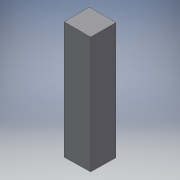
# Autodesk Inventor part: braço_junta_2
Saved by Autodesk Inventor 2018 (Build 220112000, 112)
## iProperties
Created: 2018-05-17
Part Number: braço_junta_2
Material: Genérico
Document SubType Name: Modeling
Designer: Usuario
Density: 1 g/cm^3
Appearance: Padrão
Author: Usuario
Autodesk Inventor part; units mm, degrees
ref_plane "YZ Plane" through (0, 0, 0) normal (1, 0, 0) x (0, 1, 0)
ref_plane "XZ Plane" through (0, 0, 0) normal (0, 1, 0) x (-1, 0, 0)
ref_plane "XY Plane" through (0, 0, 0) normal (0, 0, 1) x (1, 0, 0)
sketch "Esboço1" plane through (0, 0, 0) normal (0, 0, 1) x (1, 0, 0)
  line L0 (40, 339.6477) -> (0, 339.6477) projected
  line L1 (0, 339.6477) -> (40, 339.6477)
  line L2 (40, 339.6477) -> (40, 377.6477)
  line L3 (40, 377.6477) -> (0, 377.6477)
  line L4 (0, 377.6477) -> (0, 339.6477)
  line L5 (0, 377.6477) -> (65, 377.6477) construction
  point P0 (0, 0)
  dimension "d0" = 38
  constraints: 10 end point, 2 horizontal, 2 parallel, 1 perpendicular, 2 other
  measures "d0" distance of L2.end L1.end
ref_plane "Plano de trabalho1" through (-15.8286, 339.6534, -176.6311) normal (-0.0197852, 0.0122576, 0.9997291) x (0.9997606, 0.0095824, 0.0196683)
extrude "Extrusão1" add sketch "Esboço1" against normal up to surface surface through (-15.8286, 339.6534, -176.6311) normal (-0.0197852, 0.0122576, 0.9997291)
sketch "Esboço2" plane through (40, 339.6477, -175.5261) normal (0.0197852, -0.0122576, -0.9997291) x (-0.9998042, 0, -0.0197867)
  ellipse E0 centre (19.2853, 28.552) end of major axis (17.1791, 31.9526) minor radius 3.9989 construction
  ellipse E1 centre (19.2853, 9.5534) end of major axis (17.1791, 12.954) minor radius 3.9989 construction
  line L0 (40.0078, 0) -> (40.0171, 38.0029) construction
  line L1 (40.0124, 19.0014) -> (0.0046, 19.0014) construction
  line L2 (0.0092, 38.0029) -> (0, 0) construction
  line L3 (40.0171, 38.0029) -> (0.0092, 38.0029) construction
  line L4 (20.0131, 38.0029) -> (20.0039, 0) construction
  line L5 (0, 0) -> (40.0078, 0) construction
  line L6 (20.0085, 19.0014) -> (20.011, 29.0014) construction
  line L7 (20.0085, 19.0014) -> (20.0061, 9.0014) construction
  point P0 (36.5191, -341.783)
  dimension "d3" = 10
  dimension "d4" = 10
  constraints: 8 end point, 5 midpoint, 2 point on line, 2 other
  measures "d3" distance of L6.start L6.end
  measures "d4" distance of L6.start L7.end
hole "Furo1" at (20, 368.647, -176.2775) at (20, 348.6485, -176.0323) direction (-0.0197852, 0.0122576, 0.9997291) diameter 3.242 depth 10 tip angle 118 thread size "M4x0.7" class "6H" standard "ANSI Metric M Profile"
